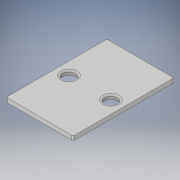
# Autodesk Inventor part: Finished_vertical stage
Saved by Autodesk Inventor 2019 (Build 230136000, 136)
## iProperties
Created: 2021-06-26
Part Number: Finished_vertical stage
Material: Generic
Document SubType Name: Modeling
Designer: 91742
Density: 1 g/cm^3
Appearance: Default
Author: 91742
Autodesk Inventor part; units mm, degrees
ref_plane "YZ Plane" through (0, 0, 0) normal (1, 0, 0) x (0, 1, 0)
ref_plane "XZ Plane" through (0, 0, 0) normal (0, 1, 0) x (-1, 0, 0)
ref_plane "XY Plane" through (0, 0, 0) normal (0, 0, 1) x (1, 0, 0)
sketch "Sketch1" plane through (0, 0, 0) normal (0, 1, 0) x (-1, 0, 0)
  line L0 (40, 60) -> (-40, 60)
  line L1 (-40, 60) -> (-40, -60)
  line L2 (-40, -60) -> (40, -60)
  line L3 (40, -60) -> (40, 60)
  line L4 (40, 60) -> (-40, -60) construction
  line L5 (-40, 60) -> (40, -60) construction
  circle A0 centre (25, 0) radius 7.5
  circle A1 centre (-25, 0) radius 7.5
  point P0 (0, 0)
  dimension "d0" = 80
  dimension "d2" = 15
  dimension "d3" = 15
  dimension "d7" = 120
  constraints: 12 end point, 2 centre point, 2 midpoint, 2 parallel, 1 horizontal, 1 perpendicular
  measures "d0" distance of L2.end L1.end
  measures "d2" diameter of A0
  measures "d3" diameter of A1
  measures "d7" distance between parallel lines of L0 L2
extrude "Extrusion1" add sketch "Sketch1" along normal blind 5
fillet "Fillet1" radius 2 6 edges at (40, 2.5, 60) (40, 2.5, -60) (-40, 2.5, -60) (-40, 2.5, 60) (-17.5, 5, 0) (32.5, 5, 0)
body "Solid1"
